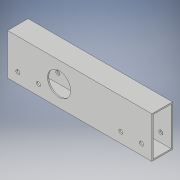
# Autodesk Inventor part: 1x2 5 in Beam Flywheel Mount
Saved by Autodesk Inventor 2018 (Build 220112000, 112)
## iProperties
Created: 2020-02-02
Part Number: 1x2 5 in Beam Flywheel Mount
Material: Generic
Document SubType Name: Modeling
Designer: Weeb No1
Density: 1 g/cm^3
Appearance: Default
Author: Weeb No1
Autodesk Inventor part; units mm, degrees
ref_plane "YZ Plane" through (0, 0, 0) normal (1, 0, 0) x (0, 1, 0)
ref_plane "XZ Plane" through (0, 0, 0) normal (0, 1, 0) x (-1, 0, 0)
ref_plane "XY Plane" through (0, 0, 0) normal (0, 0, 1) x (1, 0, 0)
sketch "Sketch1" plane through (0, 0, 0) normal (0, 0, 1) x (1, 0, 0)
  line L0 (0, 0) -> (177.8, 0)
  line L1 (177.8, 0) -> (177.8, 50.8)
  line L2 (177.8, 50.8) -> (0, 50.8)
  line L3 (0, 50.8) -> (0, 0)
  dimension "d0" = 177.8
  dimension "d1" = 50.8
  constraints: 8 end point, 2 parallel, 1 horizontal, 1 perpendicular
  measures "d0" distance of L2.end L1.end
  measures "d1" distance of L1.end L0.end
extrude "Extrusion1" add sketch "Sketch1" along normal blind 25.4
shell "Shell1" thickness 1.5875 removed faces 2 at (0, 33.8667, 16.9333) at (177.8, 16.9333, 16.9333)
sketch "Sketch2" plane through (0, 0, 25.4) normal (0, 0, 1) x (1, 0, 0)
  line L0 (0, 0) -> (63.5, 0) construction
  line L1 (63.5, 0) -> (63.5, 25.4) construction
  line L2 (63.5, 25.4) -> (0, 25.4) construction
  line L3 (0, 25.4) -> (0, 0) construction
  dimension "d5" = 63.5
  dimension "d13" = 25.4
  constraints: 8 end point, 2 parallel, 1 horizontal, 1 perpendicular
  measures "d5" distance of L2.end L1.end
  measures "d13" distance of L0.end L1.end
hole "Hole1" at (63.5, 25.4, 25.4) direction (0, 0, -1) diameter 28.575 end through all
hole "Hole2" at (12.7, 12.7, 25.4) direction (0, 0, -1) diameter 5.1594 end through all
hole "Hole3" at (38.1, 12.7, 25.4) direction (0, 0, -1) diameter 5.1594 end through all
hole "Hole4" at (165.1, 12.7, 25.4) direction (0, 0, -1) diameter 5.1594 end through all
hole "Hole5" at (139.7, 12.7, 25.4) direction (0, 0, -1) diameter 5.1594 end through all
body "Solid1"
